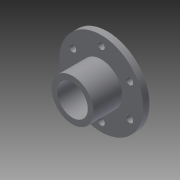
# Autodesk Inventor part: KHUB
Saved by Autodesk Inventor 2015 (Build 190159000, 159)
## iProperties
Created: 2015-01-13
Part Number: KHUB
Material: Generic
Document SubType Name: Modeling
Designer: whitaus15
Density: 1 g/cm^3
Appearance: Default
Author: whitaus15
Autodesk Inventor part; units mm, degrees
ref_plane "YZ Plane" through (0, 0, 0) normal (1, 0, 0) x (0, 1, 0)
ref_plane "XZ Plane" through (0, 0, 0) normal (0, 1, 0) x (-1, 0, 0)
ref_plane "XY Plane" through (0, 0, 0) normal (0, 0, 1) x (1, 0, 0)
sketch "Sketch1" plane through (0, 0, 0) normal (0, 0, 1) x (1, 0, 0)
  circle A0 centre (0, 0) radius 30.48
  dimension "d0" = 60.96
  constraints: 1 centre point, 1 coincident
  measures "d0" diameter of A0
extrude "Extrusion1" add sketch "Sketch1" along normal blind 4.572
sketch "Sketch2" plane through (0, 0, 4.572) normal (0, 0, 1) x (1, 0, 0)
  circle A0 centre (0, 0) radius 15.24
  dimension "d3" = 30.48
  constraints: 1 centre point, 1 coincident
  measures "d3" diameter of A0
extrude "Extrusion2" add sketch "Sketch2" along normal blind 20.828
sketch "Sketch3" plane through (0, 0, 25.4) normal (0, 0, 1) x (1, 0, 0)
  circle A0 centre (0, 0) radius 11.1125
  dimension "d6" = 22.225
  constraints: 1 centre point, 1 coincident
  measures "d6" diameter of A0
extrude "Extrusion3" cut sketch "Sketch3" against normal blind 25.4
sketch "Sketch4" plane through (0, 0, 0) normal (0, 0, -1) x (-1, 0, 0)
  circle A0 centre (0, 0) radius 23.8252
  point P0 (0, 23.8252)
  point P1 (-20.6332, 11.9126)
  point P2 (-20.6332, -11.9126)
  point P3 (0, -23.8252)
  point P4 (20.6332, -11.9126)
  point P5 (20.6332, 11.9126)
  dimension "d9" = 23.8252
  dimension "d12" = 360
  constraints: 1 coincident, 1 vertical alignment, 9 other
  measures "d9" distance of point (0, 23.825) point (0, 0)
hole "Hole1" at (0, 23.8252, 0) at (20.6332, 11.9126, 0) at (20.6332, -11.9126, 0) at (0, -23.8252, 0) at (-20.6332, -11.9126, 0) at (-20.6332, 11.9126, 0) direction (0, 0, 1) diameter 5.08 end through all
body "Solid1"
